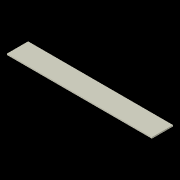
# Autodesk Inventor part: NLMFLNRMFR
Saved by Autodesk Inventor 2016 (Build 200138000, 138)
## iProperties
Created: 2017-01-21
Part Number: NLMFLNRMFR
Material: Generic
Document SubType Name: Modeling
Designer: Alexis Renderos
Density: 1 g/cm^3
Appearance: Ivory Flat
Author: Alexis Renderos
Autodesk Inventor part; units mm, degrees
ref_plane "YZ Plane" through (0, 0, 0) normal (1, 0, 0) x (0, 1, 0)
ref_plane "XZ Plane" through (0, 0, 0) normal (0, 1, 0) x (-1, 0, 0)
ref_plane "XY Plane" through (0, 0, 0) normal (0, 0, 1) x (1, 0, 0)
sketch "Sketch1" plane through (0, 0, 0) normal (0, 1, 0) x (-1, 0, 0)
  line L0 (0, -71.12) -> (0, 71.12) projected
  line L1 (-493.715, 0) -> (493.715, 0) projected
  line L2 (493.715, 0) -> (-493.715, 0) projected
  line L3 (0, -71.12) -> (0, 71.12) projected
  line L4 (352.6536, 50.8) -> (-352.6536, 50.8)
  line L5 (-352.6536, 50.8) -> (-352.6536, -50.8)
  line L6 (-352.6536, -50.8) -> (352.6536, -50.8)
  line L7 (352.6536, -50.8) -> (352.6536, 50.8)
  line L8 (352.6536, 50.8) -> (-352.6536, -50.8) construction
  line L9 (-352.6536, 50.8) -> (352.6536, -50.8) construction
  point P0 (0, 0)
  dimension "d0" = 705.3072
  dimension "d1" = 101.6
  constraints: 12 end point, 2 midpoint, 2 parallel, 1 horizontal, 1 perpendicular
  measures "d0" distance of L6.end L5.end
  measures "d1" distance of L5.end L4.end
extrude "Extrusion1" add sketch "Sketch1" along normal mid plane 6.35
body "Solid1"
